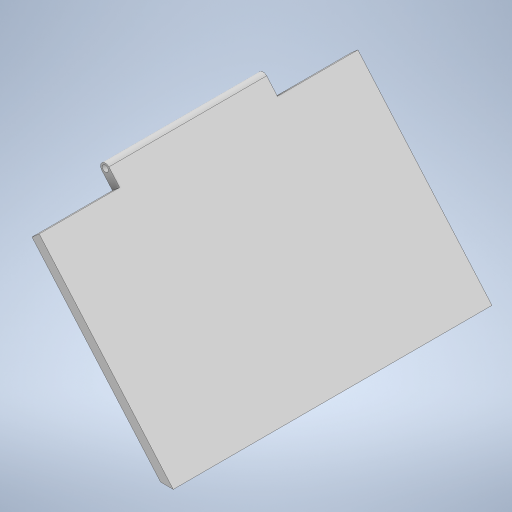
# Autodesk Inventor part: Cover2
Saved by Autodesk Inventor 2023 (Build 270158000, 158)
## iProperties
Created: 2023-03-08
Part Number: Cover2
Material: Типовые
Document SubType Name: Modeling
Designer: Josh
Density: 1 g/cm^3
Appearance: По умолчанию
Author: Josh
Autodesk Inventor part; units mm, degrees
ref_plane "YZ Plane" through (0, 0, 0) normal (1, 0, 0) x (0, 1, 0)
ref_plane "XZ Plane" through (0, 0, 0) normal (0, 1, 0) x (-1, 0, 0)
ref_plane "XY Plane" through (0, 0, 0) normal (0, 0, 1) x (1, 0, 0)
sketch "Эскиз1" plane through (0, 0, 0) normal (0, 0, 1) x (1, 0, 0)
  line L0 (0, 0) -> (-40.6757, 46.792)
  line L1 (-40.6757, 46.792) -> (-85.6757, 46.792)
  line L2 (-85.6757, 49.792) -> (-39.3085, 49.792)
  line L3 (-39.3085, 49.792) -> (3.975, 0)
  line L4 (-40.6757, 46.792) -> (-55.8266, 64.2212)
  line L5 (0, 0) -> (15.6604, 0)
  line L6 (-15.0802, 19.6341) -> (-42.5999, 51.292)
  line L7 (-85.6757, 51.292) -> (-42.5999, 51.292)
  circle A0 centre (-42.5999, 51.292) radius 1
  line L8 (-39.3085, 49.792) -> (-42.452, 53.4081)
  line L9 (-42.452, 53.4081) -> (-44.7161, 51.44)
  line L10 (-40.6757, 46.792) -> (-40.6757, 52.792)
  line L11 (-40.6757, 52.792) -> (-44.0999, 52.792)
  line L12 (-44.0999, 52.792) -> (-44.0999, 46.792)
  line L13 (-40.6757, 46.792) -> (-38.4115, 48.7602)
  line L14 (-40.3476, 46.4146) -> (-38.0835, 48.3828)
  point P0 (-59.7086, 51.292)
  dimension "d0" = 131
  dimension "d1" = 45
  dimension "d2" = 62
  dimension "d3" = 3
  dimension "d4" = 3
  dimension "d5" = 3
  dimension "d6" = 3
  dimension "d7" = 2
  dimension "d8" = 1.5
  dimension "d9" = 1.5
  dimension "d10" = 1.5
  dimension "d17" = 0.5
  constraints: 30 end point, 7 point on line, 5 perpendicular, 4 horizontal, 2 parallel, 1 centre point, 1 coincident, 1 collinear
  measures "d0" angle of L1 L0
  measures "d1" distance of L0.end L1.end
  measures "d2" distance of L0.start L0.end
  measures "d3" distance between parallel lines of L1 L2
  measures "d4" distance between parallel lines of L0 L3
  measures "d5" diameter of L0 L6
  measures "d6" diameter of L2 point (-59.709, 51.292)
  measures "d7" diameter of A0
  measures "d8" distance from line of A0.centre L9
  measures "d9" vertical distance of L10.end A0.centre
  measures "d10" distance from line of L12 A0.centre
  measures "d17" distance between parallel lines of L14 L13
extrude "Выдавливание1" add sketch "Эскиз1" along normal mid plane 49.5 contours L0 L14 L3 L5 | L0 L13 L6 L14 | L4 L2 L6 L10 | L10 L6 L13 | L6 L13 L3 L14 | L4 L12 L7 A0 L6 L2 | L10 L2 L3 L13 L6 | L6 L2 L10 | L6 A0 L7 L12 L9 L11 L8 L10 L2 | L4 L7 L12 | L10 L8 L2 | L4 L9 L12 L7 | L11 L9 L8
fillet "Сопряжение1" radius 1.5 2 edges at (-42.452, 53.4081, 0) (-44.7161, 51.44, 0)
extrude "Выдавливание2" add sketch "Эскиз1" along normal mid plane 100 contours L0 L14 L3 L5
